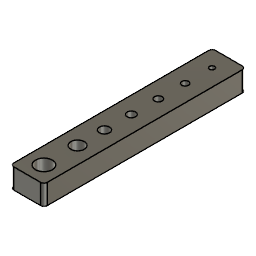
Hex key holder (Autodesk Fusion 360 design; units mm, degrees)
part number: 2026-06-27-12-15-28-567
Autodesk Fusion 360 part; units mm, degrees
sketch "Sketch1" plane through (0, 0, 0) normal (0, 0, 1) x (1, 0, 0)
  line L0 (10, -60) -> (-10, -60)
  line L1 (-10, -60) -> (-10, 60)
  line L2 (-10, 60) -> (10, 60)
  line L3 (10, 60) -> (10, -60)
  line L4 (10, -60) -> (-10, 60) construction
  line L5 (-10, -60) -> (10, 60) construction
  dimension "d1" = 20
  dimension "d2" = 120
  constraint horizontal L0
  constraint perpendicular L0 L1
  constraint parallel L0 L2
  constraint parallel L1 L3
  constraint coincident L4 origin
  constraint coincident L5 origin
  measures "d1" distance of L1.end L2.end
  measures "d2" distance of L0.end L1.end
extrude "Extrude1" add sketch "Sketch1" along normal blind 12
sketch "Sketch2" plane through (0, 0, 12) normal (0, 0, 1) x (-1, 0, 0)
  line L0 (-10, -60) -> (10, -60)
  line L1 (10, -60) -> (10, 60)
  line L2 (10, 60) -> (-10, 60)
  line L3 (-10, 60) -> (-10, -60)
  circle A0 centre (0, -50) radius 2
  circle A1 centre (0, 50) radius 2
extrude "Extrude2" cut sketch "Sketch2" against normal blind 12 contours A0
sketch "Sketch3" plane through (0, 0, 12) normal (0, 0, 1) x (-1, 0, 0)
  circle A0 centre (0, -50) radius 2
  line L0 (-10, -60) -> (10, -60)
  line L1 (10, -60) -> (10, 60)
  line L2 (10, 60) -> (-10, 60)
  line L3 (-10, 60) -> (-10, -60)
  circle A1 centre (0, 50) radius 2
  dimension "d10" = 4
  measures "d10" diameter of A1
extrude "Extrude3" cut sketch "Sketch3" against normal blind 12 contours A1
sketch "Sketch4" plane through (0, 0, 12) normal (0, 0, 1) x (-1, 0, 0)
  circle A0 centre (0, 50) radius 2
  circle A1 centre (0, -50) radius 2
  line L0 (-10, -60) -> (10, -60)
  line L1 (10, -60) -> (10, 60)
  line L2 (10, 60) -> (-10, 60)
  line L3 (-10, 60) -> (-10, -60)
  circle A2 centre (0, -34) radius 2
  circle A3 centre (0, -18) radius 2
  circle A4 centre (0, -2) radius 2
  circle A5 centre (0, 14) radius 2
  circle A6 centre (0, 30) radius 2
  point P0 (0, -34)
  point P1 (0, -18)
  point P2 (0, -2)
  point P3 (0, 14)
  point P4 (0, 30)
  point P5 (0, -18)
  point P6 (0, -2)
  point P7 (0, 14)
  point P8 (0, 30)
  point P9 (0, 46)
  dimension "d15" = 0
  dimension "d16" = 80
  dimension "d19" = 0
  dimension "d20" = 80
extrude "Extrude4" cut sketch "Sketch4" against normal blind 12 contours A2 | A3 | A4 | A5 | A6
sketch "Sketch5" plane through (0, 0, 12) normal (0, 0, 1) x (-1, 0, 0)
  line L0 (-10, -60) -> (10, -60)
  line L1 (10, -60) -> (10, 60)
  line L2 (10, 60) -> (-10, 60)
  line L3 (-10, 60) -> (-10, -60)
  circle A0 centre (0, -50) radius 2
  circle A1 centre (0, 50) radius 2
  circle A2 centre (0, 30) radius 2
  circle A3 centre (0, -34) radius 2
  circle A4 centre (0, 14) radius 2
  circle A5 centre (0, -18) radius 2
  circle A6 centre (0, -2) radius 2
sketch "Sketch6" plane through (0, 0, 12) normal (0, 0, 1) x (1, 0, 0)
  circle A0 centre (0, 50) radius 1.5
  circle A1 centre (0, 18) radius 2.25
  circle A2 centre (0, 2) radius 2.5
  circle A3 centre (0, -14) radius 3
  circle A4 centre (0, -30) radius 4
  circle A5 centre (0, -50) radius 5
  dimension "d26" = 3
  dimension "d27" = 4.5
  dimension "d28" = 5
  dimension "d29" = 6
  dimension "d30" = 8
  dimension "d31" = 10
  measures "d26" diameter of A0
  measures "d27" diameter of A1
  measures "d28" diameter of A2
  measures "d29" diameter of A3
  measures "d30" diameter of A4
  measures "d31" diameter of A5
extrude "Extrude5" add sketch "Sketch5" against normal blind 12 contours A0
extrude "Extrude6" add sketch "Sketch6" along normal blind 12 contours A0
extrude "Extrude7" cut 1 faces at (-0.1827, 50.4654, 24) along direction (0, 0, -1) blind 12
sketch "Sketch7" plane through (0, 0, 12) normal (0, 0, 1) x (-1, 0, 0)
  line L0 (-10, -60) -> (10, -60)
  line L1 (10, -60) -> (10, 60)
  line L2 (10, 60) -> (-10, 60)
  line L3 (-10, 60) -> (-10, -60)
  circle A0 centre (0, 50) radius 2
  circle A1 centre (0, 30) radius 2
  circle A2 centre (0, -34) radius 2
  circle A3 centre (0, 14) radius 2
  circle A4 centre (0, -18) radius 2
  circle A5 centre (0, -2) radius 2
  circle A6 centre (0, -50) radius 1.5
  dimension "d38" = 3
  measures "d38" diameter of A6
extrude "Extrude8" cut sketch "Sketch7" against normal blind 12 contours A6
sketch "Sketch8" plane through (0, 0, 12) normal (0, 0, 1) x (-1, 0, 0)
  circle A0 centre (0, -50) radius 1.5
  line L0 (-10, -60) -> (10, -60)
  line L1 (10, -60) -> (10, 60)
  line L2 (10, 60) -> (-10, 60)
  line L3 (-10, 60) -> (-10, -60)
  circle A1 centre (0, 50) radius 2
  circle A2 centre (0, 30) radius 2
  circle A3 centre (0, -34) radius 2
  circle A4 centre (0, 14) radius 2
  circle A5 centre (0, -18) radius 2
  circle A6 centre (0, -2) radius 2
  circle A7 centre (0, -18) radius 2.25
  circle A8 centre (0, -2) radius 2.5
  circle A9 centre (0, 14) radius 3
  circle A10 centre (0, 30) radius 4
  circle A11 centre (0, 50) radius 5
  dimension "d41" = 4.5
  dimension "d42" = 5
  dimension "d43" = 6
  dimension "d44" = 8
  dimension "d45" = 10
  constraint concentric A5 A7
  constraint concentric A6 A8
  constraint concentric A4 A9
  constraint concentric A2 A10
  constraint concentric A1 A11
  measures "d41" diameter of A7
  measures "d42" diameter of A8
  measures "d43" diameter of A9
  measures "d44" diameter of A10
  measures "d45" diameter of A11
extrude "Extrude9" cut sketch "Sketch8" against normal blind 12 contours A11
sketch "Sketch9" plane through (0, 0, 12) normal (0, 0, 1) x (-1, 0, 0)
  circle A0 centre (0, -2) radius 2
  circle A1 centre (0, -18) radius 2
  circle A2 centre (0, 14) radius 2
  circle A3 centre (0, -34) radius 2
  circle A4 centre (0, 30) radius 2
  line L0 (-10, -60) -> (10, -60)
  line L1 (10, -60) -> (10, 60)
  line L2 (10, 60) -> (-10, 60)
  line L3 (-10, 60) -> (-10, -60)
  circle A5 centre (0, -50) radius 1.5
  circle A6 centre (0, 50) radius 5
  circle A7 centre (0, 30) radius 4
  dimension "d48" = 8
  constraint concentric A4 A7
  measures "d48" diameter of A7
extrude "Extrude10" cut sketch "Sketch9" against normal blind 12 contours A7
sketch "Sketch10" plane through (0, 0, 12) normal (0, 0, 1) x (-1, 0, 0)
  circle A0 centre (0, 50) radius 5
  circle A1 centre (0, -50) radius 1.5
  line L0 (-10, -60) -> (10, -60)
  line L1 (10, -60) -> (10, 60)
  line L2 (10, 60) -> (-10, 60)
  line L3 (-10, 60) -> (-10, -60)
  circle A2 centre (0, -34) radius 2
  circle A3 centre (0, 14) radius 2
  circle A4 centre (0, -18) radius 2
  circle A5 centre (0, -2) radius 2
  circle A6 centre (0, 30) radius 4
  circle A7 centre (0, 14) radius 3
  dimension "d51" = 6
  constraint concentric A3 A7
  measures "d51" diameter of A7
extrude "Extrude11" cut sketch "Sketch10" against normal blind 12 contours A7
sketch "Sketch11" plane through (0, 0, 12) normal (0, 0, 1) x (-1, 0, 0)
  circle A0 centre (0, 30) radius 4
  circle A1 centre (0, -2) radius 2
  circle A2 centre (0, -18) radius 2
  circle A3 centre (0, -34) radius 2
  line L0 (-10, -60) -> (10, -60)
  line L1 (10, -60) -> (10, 60)
  line L2 (10, 60) -> (-10, 60)
  line L3 (-10, 60) -> (-10, -60)
  circle A4 centre (0, -50) radius 1.5
  circle A5 centre (0, 50) radius 5
  circle A6 centre (0, 14) radius 3
  circle A7 centre (0, -2) radius 2.5
  dimension "d54" = 5
  constraint concentric A1 A7
  measures "d54" diameter of A7
extrude "Extrude12" cut sketch "Sketch11" against normal blind 12 contours A7
sketch "Sketch12" plane through (0, 0, 12) normal (0, 0, 1) x (-1, 0, 0)
  circle A0 centre (0, 14) radius 3
  circle A1 centre (0, 50) radius 5
  circle A2 centre (0, -50) radius 1.5
  line L0 (-10, -60) -> (10, -60)
  line L1 (10, -60) -> (10, 60)
  line L2 (10, 60) -> (-10, 60)
  line L3 (-10, 60) -> (-10, -60)
  circle A3 centre (0, -34) radius 2
  circle A4 centre (0, -18) radius 2
  circle A5 centre (0, 30) radius 4
  circle A6 centre (0, -2) radius 2.5
  circle A7 centre (0, -18) radius 2.25
  dimension "d57" = 4.5
  constraint concentric A4 A7
  measures "d57" diameter of A7
extrude "Extrude13" cut sketch "Sketch12" against normal blind 12 contours A7
fillet "Fillet1" radius 2 4 edges at (-10, -60, 6) (-10, 60, 6) (10, 60, 6) (10, -60, 6)
